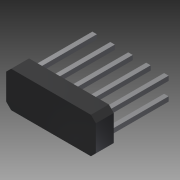
# Autodesk Inventor part: connecteur 10
Saved by Autodesk Inventor 2014 SP2 (Build 180246200, 246)
## iProperties
Created: 2015-03-18
Part Number: connecteur 10
Material: Générique
Document SubType Name: Modeling
Designer: sd
Density: 1 g/cm^3
Appearance: Par défaut
Author: sd
Autodesk Inventor part; units mm, degrees
ref_plane "YZ Plane" through (0, 0, 0) normal (1, 0, 0) x (0, 1, 0)
ref_plane "XZ Plane" through (0, 0, 0) normal (0, 1, 0) x (-1, 0, 0)
ref_plane "XY Plane" through (0, 0, 0) normal (0, 0, 1) x (1, 0, 0)
sketch "Esquisse1" plane through (0, 0, 0) normal (0, 1, 0) x (-1, 0, 0)
  line L0 (-6.35, 2.54) -> (6.35, 2.54)
  line L1 (6.35, 2.54) -> (6.35, -2.54)
  line L2 (6.35, -2.54) -> (-6.35, -2.54)
  line L3 (-6.35, -2.54) -> (-6.35, 2.54)
  point P0 (0, 0)
  dimension "d0" = 12.7
  dimension "d1" = 5.08
  dimension "d2" = 6.35
  dimension "d3" = 2.54
  constraints: 8 end point, 2 parallel, 1 horizontal, 1 perpendicular
  measures "d0" distance of L0.start L0.end
  measures "d1" distance of L2.end L0.start
  measures "d2" horizontal distance of point (0, 0) L0.start
  measures "d3" vertical distance of point (0, 0) L0.start
extrude "Extrusion1" add sketch "Esquisse1" along normal blind 2.54
chamfer "Chanfrein1" distance 0.7 angle 45 4 edges at (6.35, 1.27, 2.54) (6.35, 1.27, -2.54) (-6.35, 1.27, -2.54) (-6.35, 1.27, 2.54)
sketch "Esquisse2" plane through (0, 2.54, 0) normal (0, 1, 0) x (1, 0, 0)
  line L0 (5.65, 2.54) -> (-5.65, 2.54) projected
  line L1 (-6.35, 1.84) -> (-6.35, -1.84) projected
  line L2 (-5.08, 1.27) -> (-4.44, 1.27)
  line L3 (-4.44, 1.27) -> (-4.44, 0.63)
  line L4 (-4.44, 0.63) -> (-5.08, 0.63)
  line L5 (-5.08, 0.63) -> (-5.08, 1.27)
  point P0 (0, 0)
  dimension "d9" = 0.64
  dimension "d10" = 0.64
  dimension "d11" = 1.27
  dimension "d12" = 1.27
  constraints: 8 end point, 2 parallel, 1 horizontal, 1 perpendicular
  measures "d9" distance of L2.start L2.end
  measures "d10" distance of L4.end L2.start
  measures "d11" distance between parallel lines of L1 L5
  measures "d12" distance between parallel lines of L0 L2
extrude "Extrusion2" add sketch "Esquisse2" along normal blind 8.5
pattern_linear "Réseau rectangulaire1" count 5 spacing 2.54 along (1, 0, 0) count 2 spacing 2.54 along (0, 0, 1) of "Extrusion2"
chamfer "Chanfrein2" distance 0.1 angle 45 40 edges at (-4.76, 11.04, -0.63) (-4.44, 11.04, -0.95) (-4.76, 11.04, -1.27) (-5.08, 11.04, -0.95) (-2.22, 11.04, -0.63) (-2.54, 11.04, -0.95) (-1.9, 11.04, -0.95) (-2.22, 11.04, -1.27) (0, 11.04, -0.95) (0.32, 11.04, -0.63) (0.64, 11.04, -0.95) (0.32, 11.04, -1.27) (0.32, 11.04, 1.27) (0.64, 11.04, 1.59) (0.32, 11.04, 1.91) (0, 11.04, 1.59) (-1.9, 11.04, 1.59) (-2.22, 11.04, 1.27) (-2.22, 11.04, 1.91) (-2.54, 11.04, 1.59) (-5.08, 11.04, 1.59) (-4.76, 11.04, 1.27) (-4.44, 11.04, 1.59) (-4.76, 11.04, 1.91) (2.54, 11.04, -0.95) (3.18, 11.04, -0.95) (2.86, 11.04, -0.63) (2.86, 11.04, -1.27) (2.86, 11.04, 1.27) (3.18, 11.04, 1.59) (2.86, 11.04, 1.91) (2.54, 11.04, 1.59) (5.08, 11.04, 1.59) (5.4, 11.04, 1.91) (5.72, 11.04, 1.59) (5.4, 11.04, 1.27) (5.4, 11.04, -0.63) (5.08, 11.04, -0.95) (5.4, 11.04, -1.27) (5.72, 11.04, -0.95)
equation "\"d2\" = 0.5 * d0"
equation "\"d3\" = 0.5 * d1"
equation "\"d10\" = d9"
